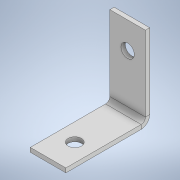
# Autodesk Inventor part: 4.5x1
Saved by Autodesk Inventor 2020 (Build 240168000, 168)
## iProperties
Created: 2019-11-19
Part Number: 4.5x1
Material: Generic
Document SubType Name: Sheet Metal
Designer: ellio
Density: 1 g/cm^3
Sheet Metal Rule: Default
Appearance: Default
Author: ellio
Autodesk Inventor part; units mm, degrees
ref_plane "YZ Plane" through (0, 0, 0) normal (1, 0, 0) x (0, 1, 0)
ref_plane "XZ Plane" through (0, 0, 0) normal (0, 1, 0) x (-1, 0, 0)
ref_plane "XY Plane" through (0, 0, 0) normal (0, 0, 1) x (1, 0, 0)
sketch "Sketch1" plane through (0, 0, 0) normal (0, 1, 0) x (-1, 0, 0)
  line L0 (0, 0) -> (25.4, 0)
  line L1 (25.4, 0) -> (25.4, -114.3)
  line L2 (25.4, -114.3) -> (0, -114.3)
  line L3 (0, -114.3) -> (0, 0)
  circle A0 centre (12.7, -19.05) radius 4.7625
  circle A1 centre (12.7, -95.25) radius 4.7625
  dimension "d0" = 25.4
  dimension "d1" = 114.3
  dimension "d2" = 9.525
  dimension "d3" = 9.525
  measures "d0" distance of L1.end L2.end
  measures "d1" distance of L0.end L1.end
  measures "d2" diameter of A0
  measures "d3" diameter of A1
extrude "Plate1" add sketch "Sketch1" along normal blind 3.048
sketch "Sketch2" plane through (0, 3.048, 0) normal (0, 1, 0) x (1, 0, 0)
  line L0 (-25.4, 0) -> (-25.4, 114.3) projected
  line L1 (-25.4, 57.15) -> (0, 57.15)
  point P0 (0, 0)
  constraints: 2 end point, 1 horizontal, 1 midpoint
fold "Fold1" angle 90 bend radius 3.048 thickness 3.048 k factor 0.44 line from (-25.4, 3.048, -57.15) to (0, 3.048, -57.15) line at bend centre moving side (0, 0, -1) folds toward (0, 1, 0)
equation "\"d4\" = Thickness"
equation "\"d5\" = BendReliefWidth"
equation "\"d6\" = BendReliefDepth"
equation "\"d7\" = MinimumRemnant"
equation "\"d8\" = TransitionRadius"
equation "\"d10\" = BendRadius"
equation "\"BendRadius\" = Thickness"
equation "\"BendReliefWidth\" = Thickness"
equation "\"BendReliefDepth\" = 0.5 * Thickness"
equation "\"CornerReliefSize\" = 4 * Thickness"
equation "\"MinimumRemnant\" = 2 * Thickness"
equation "\"TransitionRadius\" = BendRadius"
equation "\"JacobiRadiusSize\" = BendRadius"
equation "\"GapSize\" = Thickness"
equation "\"Thickness\" = 3.048"
body "Solid1"
